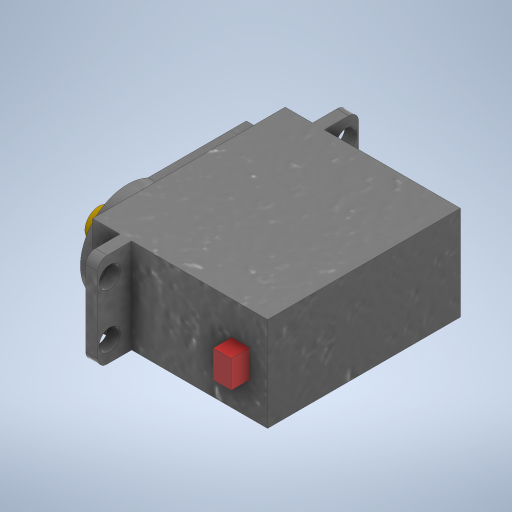
# Autodesk Inventor part: ServoMotor
Saved by Autodesk Inventor 2024 (Build 280153000, 153)
## iProperties
Created: 2024-01-04
Part Number: ServoMotor
Material: Genérico
Document SubType Name: Modeling
Designer: sergi
Density: 1 g/cm^3
Appearance: Valor por defecto
Author: sergi
Autodesk Inventor part; units mm, degrees
ref_plane "YZ Plane" through (0, 0, 0) normal (1, 0, 0) x (0, 1, 0)
ref_plane "XZ Plane" through (0, 0, 0) normal (0, 1, 0) x (-1, 0, 0)
ref_plane "XY Plane" through (0, 0, 0) normal (0, 0, 1) x (1, 0, 0)
sketch "Boceto1" plane through (0, 0, 0) normal (0, 1, 0) x (-1, 0, 0)
  line L0 (0, 0) -> (36.8, 0)
  line L1 (36.8, 0) -> (36.8, -40.5)
  line L2 (36.8, -40.5) -> (0, -40.5)
  line L3 (0, -40.5) -> (0, 0)
  line L4 (0, -40.5) -> (28.55, -40.5)
  line L5 (28.55, -40.5) -> (28.55, -47.65)
  line L6 (28.55, -47.65) -> (31.05, -47.65)
  line L7 (31.05, -47.65) -> (31.05, -40.5)
  line L8 (28.55, 0) -> (28.55, 7.15)
  line L9 (28.55, 7.15) -> (31.05, 7.15)
  line L10 (31.05, 7.15) -> (31.05, 0)
  dimension "d0" = 36.8
  dimension "d1" = 40.5
  dimension "d2" = 28.55
  dimension "d3" = 7.15
  dimension "d4" = 2.5
  dimension "d5" = 7.15
  dimension "d6" = 2.5
  constraints: 22 end point, 6 perpendicular, 4 point on line, 2 parallel, 1 horizontal, 1 vertical
  measures "d0" distance of L1.end L2.end
  measures "d1" distance of L0.end L1.end
  measures "d2" distance of L2.end L4.end
  measures "d3" distance of L4.end L5.end
  measures "d4" distance of L5.end L6.end
  measures "d5" distance of L8.start L8.end
  measures "d6" distance of L8.end L9.end
extrude "Extrusión1" add sketch "Boceto1" along normal blind 19.8
sketch "Boceto2" plane through (-36.8, 0, -40.5) normal (-1, 0, 0) x (0, 0, 1)
  line L0 (0, 0) -> (40.5, 0) projected
  line L1 (40.5, 0) -> (40.5, 19.8) projected
  line L2 (0, 19.8) -> (40.5, 19.8) projected
  line L3 (0, 0) -> (0, 19.8) projected
  line L4 (0, 0) -> (5.65, 0)
  line L5 (40.5, 18.85) -> (40.5, 0.95)
  line L6 (26.3683, 0.95) -> (5.65, 0.95)
  line L7 (40.5, 0) -> (40.5, 19.8) projected
  line L8 (40.5, 9.9) -> (30.6, 9.9)
  arc A0 (26.3683, 0.95) -> (26.3683, 18.85) centre (30.6, 9.9) ccw
  arc A1 (5.65, 14.48) -> (5.65, 5.32) centre (9.7412, 9.9) ccw
  line L9 (5.65, 18.85) -> (26.3683, 18.85)
  line L10 (5.65, 0.95) -> (5.65, 5.32)
  line L11 (5.65, 14.48) -> (5.65, 18.85)
  line L12 (5.65, 0.95) -> (5.65, 5.32)
  line L13 (5.65, 14.48) -> (5.65, 18.85)
  point P0 (5.65, 0.95)
  dimension "d11" = 17.9
  dimension "d12" = 9.9
  constraints: 18 end point, 5 point on circle, 4 parallel, 2 centre point, 2 point on line, 1 coincident, 1 horizontal, 1 midpoint, 1 perpendicular
  measures "d11" distance of L10.start L9.start
  measures "d12" distance of L8.start L8.end
extrude "Extrusión2" add sketch "Boceto2" along normal blind 2.52 contours A0 L6 L10 A1 L11 L9
sketch "Boceto3" plane through (-39.32, 0, -40.5) normal (-1, 0, 0) x (0, 0, 1)
  arc A0 (26.3683, 0.95) -> (26.3683, 18.85) centre (30.6, 9.9) ccw projected
  line L0 (26.3683, 18.85) -> (5.65, 18.85) projected
  line L1 (5.65, 18.85) -> (5.65, 14.48) projected
  arc A1 (5.65, 14.48) -> (5.65, 5.32) centre (9.7412, 9.9) ccw projected
  line L2 (5.65, 5.32) -> (5.65, 0.95) projected
  line L3 (5.65, 0.95) -> (26.3683, 0.95) projected
  circle A2 centre (30.6, 9.9) radius 6.575
  point P0 (40.5, 0)
  dimension "d18" = 13.15
  constraints: 1 centre point, 1 coincident
  measures "d18" diameter of A2
extrude "Extrusión3" add sketch "Boceto3" along normal blind 2.15 contours A2
sketch "Boceto4" plane through (-41.47, 9.9, -9.9) normal (-1, 0, 0) x (0, 0, 1)
  circle A0 centre (0, 0) radius 6.575 projected
  circle A1 centre (0, 0) radius 2.9
  point P0 (9.9, -9.9)
  dimension "d21" = 5.8
  constraints: 1 centre point, 1 coincident
  measures "d21" diameter of A1
extrude "Extrusión4" add sketch "Boceto4" along normal blind 3.9 contours A1
sketch "Boceto5" plane through (-45.37, 9.9, -9.9) normal (-1, 0, 0) x (0, 0, 1)
  circle A0 centre (0, 0) radius 2.9 projected
  point P0 (9.9, -9.9)
  constraints: 1 coincident
hole "Agujero1" at (-45.37, 9.9, -9.9) direction (1, 0, 0) diameter 2.6 depth 10 tip angle 118
sketch "Boceto6" plane through (-28.55, 0, 0) normal (0, 0, 1) x (1, 0, 0)
  line L0 (0, 0) -> (28.55, 0) projected
  line L1 (28.55, 0) -> (28.55, 19.8) projected
  line L2 (0, 19.8) -> (28.55, 19.8) projected
  line L3 (0, 0) -> (0, 19.8) projected
  line L4 (21, 9.9) -> (21, 12.8)
  line L5 (21, 12.8) -> (24.8, 12.8)
  line L6 (24.8, 12.8) -> (24.8, 7)
  line L7 (24.8, 7) -> (21, 7)
  line L8 (21, 7) -> (21, 12.8)
  line L9 (24.8, 12.8) -> (28.55, 12.8)
  dimension "d34" = 2.9
  dimension "d35" = 5.8
  constraints: 12 end point, 2 parallel, 2 perpendicular, 1 horizontal, 1 point on line
  measures "d34" distance of L4.start L4.end
  measures "d35" distance of L5.end L6.end
extrude "Extrusión5" add sketch "Boceto6" along normal blind 3.9 contours L4 L5 L6 L7 L8
sketch "Boceto7" plane through (-31.05, 0, 0) normal (-1, 0, 0) x (0, 0, 1)
  line L0 (0, 0) -> (7.15, 0) projected
  line L1 (7.15, 0) -> (7.15, 19.8) projected
  line L2 (0, 19.8) -> (7.15, 19.8) projected
  line L3 (0, 0) -> (0, 19.8) projected
  line L4 (0, 0) -> (2.26, 0)
  line L5 (2.26, 0) -> (2.26, 19.8)
  line L6 (7.15, 9.9) -> (0, 9.9)
  line L7 (7.15, 10.4) -> (0, 10.4)
  line L8 (7.15, 9.4) -> (0, 9.4)
  point P0 (0, 0)
  point P1 (0, 10.4)
  point P2 (0, 9.4)
  dimension "d38" = 2.26
  dimension "d39" = 0.5
  dimension "d40" = 0.5
  constraints: 10 end point, 2 midpoint, 2 parallel, 2 point on line, 1 perpendicular
  measures "d38" distance of L0.start L4.end
  measures "d39" distance between parallel lines of L6 L7
  measures "d40" distance between parallel lines of L6 L8
extrude "Extrusión6" add sketch "Boceto7" along normal blind 1.35 contours L3 L6 L5 L8 | L5 L6 L1 L8 | L3 L7 L5 L6 | L5 L7 L1 L6
chamfer "Chaflán1" distance 6 distance2 1.35 1 edges at (-32.4, 9.9, 7.15) measured on face at (-32.4, 9.9, 6.65)
fillet "Empalme1" radius 2 2 edges at (-29.8, 0, 7.15) (-29.8, 19.8, 7.15)
sketch "Boceto8" plane through (-31.05, 0, 0) normal (-1, 0, 0) x (0, 0, 1)
  arc A0 (5.15, 0) -> (7.15, 2) centre (5.15, 2) ccw projected
  line L0 (7.15, 2) -> (7.15, 9.4) projected
  line L1 (7.15, 9.4) -> (0, 9.4) projected
  line L2 (0, 0) -> (0, 9.4) projected
  line L3 (0, 0) -> (5.15, 0) projected
  line L4 (3.575, 0) -> (3.575, 2)
  line L5 (3.575, 2) -> (3.575, 6.4)
  line L6 (0, 0) -> (2.4, 0)
  line L7 (2.4, 0) -> (2.4, 4.2)
  line L8 (2.4, 4.2) -> (4.6, 4.2)
  circle A1 centre (4.6, 4.2) radius 2.2
  arc A2 (7.15, 17.8) -> (5.15, 19.8) centre (5.15, 17.8) ccw projected
  line L9 (0, 19.8) -> (5.15, 19.8) projected
  line L10 (0, 10.4) -> (0, 19.8) projected
  line L11 (0, 10.4) -> (7.15, 10.4) projected
  line L12 (7.15, 10.4) -> (7.15, 17.8) projected
  line L13 (4.6, 4.2) -> (4.6, 19.8)
  line L14 (4.6, 19.8) -> (4.6, 15.6)
  circle A3 centre (4.6, 15.6) radius 2.2
  point P0 (0, 0)
  dimension "d47" = 2
  dimension "d48" = 4.4
  dimension "d49" = 2.4
  dimension "d50" = 2.2
  dimension "d58" = 4.2
  dimension "d59" = 4.4
  constraints: 14 end point, 5 point on line, 2 coincident, 2 perpendicular, 2 vertical, 1 centre point, 1 horizontal alignment, 2 other
  measures "d47" distance of L4.start L4.end
  measures "d48" distance of L4.end L5.end
  measures "d49" distance of L2.start L6.end
  measures "d50" distance of L7.end L8.end
  measures "d58" distance of L13.end L14.end
  measures "d59" diameter of A3
hole "Agujero2" at (-31.05, 4.2, 4.6) at (-31.05, 15.6, 4.6) direction (1, 0, 0) diameter 4.4 depth 10 tip angle 118
ref_plane "Plano de trabajo1" through (-28.55, 0, -20.25) normal (0, 0, 1) x (1, 0, 0)
mirror "Simetría1" about plane through (-28.55, 0, -20.25) normal (0, 0, 1) of "Extrusión6", "Agujero2"
chamfer "Chaflán2" distance 6 distance2 1.35 1 edges at (-32.4, 9.9, -47.65) measured on face at (-32.4, 9.9, -47.15)
fillet "Empalme2" radius 2 2 edges at (-29.8, 0, -47.65) (-29.8, 19.8, -47.65)
